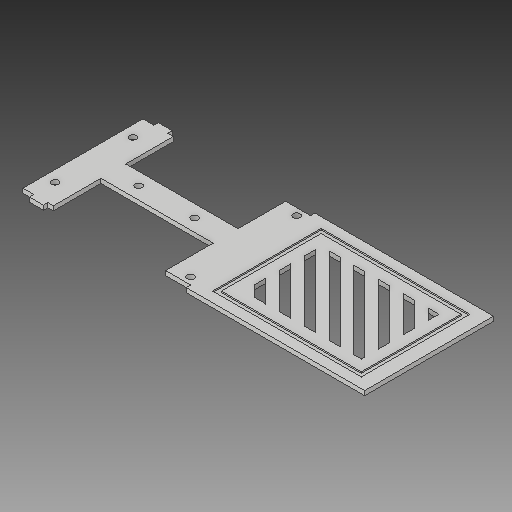
# Autodesk Inventor part: cuerpo-base-bateria
Saved by Autodesk Inventor 2019 (Build 230136000, 136)
## iProperties
Created: 2020-03-02
Part Number: cuerpo-base-bateria
Material: Generic
Document SubType Name: Modeling
Designer: jacqu
Density: 1 g/cm^3
Appearance: Default
ancho_acople_hombros: 86.662 mm
largo_abdomen_robot: 146.950 mm
Author: jacqu
Autodesk Inventor part; units mm, degrees
ref_plane "YZ Plane" through (0, 0, 0) normal (1, 0, 0) x (0, 1, 0)
ref_plane "XZ Plane" through (0, 0, 0) normal (0, 1, 0) x (-1, 0, 0)
ref_plane "XY Plane" through (0, 0, 0) normal (0, 0, 1) x (1, 0, 0)
sketch "Sketch9" plane through (0, 0, 0) normal (0, 1, 0) x (-1, 0, 0)
  line L0 (0, 0) -> (-250, 0)
  line L1 (-250, 0) -> (-250, -86.6623)
  line L2 (-250, -86.6623) -> (0, -86.6623)
  line L3 (0, -86.6623) -> (0, 0)
  dimension "d59" = 86.6623
  dimension "d60" = 250
  constraints: 8 end point, 2 parallel, 1 horizontal, 1 perpendicular
  measures "d59" distance of L2.end L0.start
  measures "d60" distance between parallel lines of L3 L1
extrude "Extrusion5" add sketch "Sketch9" along normal blind 3.2
sketch "Sketch10" plane through (0, 3.2, 0) normal (0, 1, 0) x (1, 0, 0)
  line L0 (22, 0) -> (103.05, 0)
  line L1 (103.05, 0) -> (103.05, 34.3311)
  line L2 (103.05, 34.3311) -> (22, 34.3311)
  line L3 (22, 34.3311) -> (22, 0)
  line L4 (250, 86.6623) -> (0, 86.6623) projected
  line L5 (103.05, 86.6623) -> (22, 86.6623)
  line L6 (22, 86.6623) -> (22, 52.3311)
  line L7 (22, 52.3311) -> (103.05, 52.3311)
  line L8 (103.05, 52.3311) -> (103.05, 86.6623)
  line L9 (0, 0) -> (250, 0) projected
  line L10 (0, 86.6623) -> (0, 0) projected
  dimension "d63" = 22
  dimension "d64" = 34.3311
  dimension "d65" = 81.05
  dimension "d66" = 34.3311
  constraints: 16 end point, 4 parallel, 4 point on line, 2 horizontal, 2 perpendicular
  measures "d63" distance between parallel lines of L10 L3
  measures "d64" distance of L2.end L0.start
  measures "d65" distance between parallel lines of L3 L1
  measures "d66" distance between parallel lines of L4 L7
extrude "Extrusion6" cut sketch "Sketch10" against normal blind 3.2
sketch "Sketch11" plane through (0, 3.2, 0) normal (0, 1, 0) x (1, 0, 0)
  line L0 (237.05, 7.3311) -> (136.05, 7.3311)
  line L1 (136.05, 7.3311) -> (136.05, 79.3311)
  line L2 (136.05, 79.3311) -> (237.05, 79.3311)
  line L3 (237.05, 79.3311) -> (237.05, 7.3311)
  line L4 (103.05, 86.6623) -> (103.05, 52.3311) projected
  line L5 (0, 86.6623) -> (0, 0) projected
  line L6 (103.05, 0) -> (250, 0) projected
  line L7 (121.05, 0) -> (121.05, 86.188) construction
  line L8 (103.05, 34.3311) -> (103.05, 0) projected
  line L9 (240.25, 4.1311) -> (132.85, 4.1311)
  line L10 (132.85, 4.1311) -> (132.85, 82.5311)
  line L11 (132.85, 82.5311) -> (240.25, 82.5311)
  line L12 (240.25, 82.5311) -> (240.25, 4.1311)
  dimension "d69" = 72
  dimension "d70" = 101
  dimension "d71" = 33
  dimension "d72" = 86.6623
  dimension "d73" = 7.3311
  dimension "d74" = 18
  dimension "d75" = 3.2
  dimension "d76" = 3.2
  dimension "d77" = 3.2
  dimension "d78" = 3.2
  constraints: 18 end point, 4 parallel, 2 horizontal, 2 perpendicular, 1 point on line, 1 vertical
  measures "d69" distance of L2.end L0.start
  measures "d70" distance of L1.end L2.end
  measures "d71" distance between parallel lines of L4 L1
  measures "d72" distance of L5.start L5.end
  measures "d73" distance between parallel lines of L6 L0
  measures "d74" distance between parallel lines of L7 L8
  measures "d75" distance between parallel lines of L3 L12
  measures "d76" distance between parallel lines of L9 L0
  measures "d77" distance between parallel lines of L11 L2
  measures "d78" distance between parallel lines of L10 L1
extrude "Extrusion7" cut sketch "Sketch11" against normal blind 1
sketch "Sketch12" plane through (0, 3.2, 0) normal (0, 1, 0) x (1, 0, 0)
  line L0 (237.05, 7.3311) -> (237.05, 79.3311) projected
  line L1 (237.05, 79.3311) -> (136.05, 79.3311) projected
  line L2 (136.05, 79.3311) -> (136.05, 7.3311) construction
  line L3 (136.05, 7.3311) -> (237.05, 7.3311) projected
  line L4 (144.05, 15.3311) -> (229.05, 15.3311) construction
  line L5 (229.05, 15.3311) -> (229.05, 71.3311) construction
  line L6 (229.05, 71.3311) -> (144.05, 71.3311) construction
  line L7 (144.05, 71.3311) -> (144.05, 15.3311) construction
  line L8 (152.05, 15.3311) -> (144.05, 23.3311)
  line L9 (144.05, 23.3311) -> (144.05, 31.3311)
  line L10 (144.05, 31.3311) -> (160.05, 15.3311)
  line L11 (160.05, 15.3311) -> (152.05, 15.3311)
  line L12 (169.9495, 15.3311) -> (144.05, 41.2306)
  line L13 (144.05, 41.2306) -> (144.05, 49.2306)
  line L14 (144.05, 49.2306) -> (177.9495, 15.3311)
  line L15 (169.9495, 15.3311) -> (177.9495, 15.3311)
  line L16 (187.849, 15.3311) -> (144.05, 59.1301)
  line L17 (144.05, 59.1301) -> (144.05, 67.1301)
  line L18 (144.05, 67.1301) -> (195.849, 15.3311)
  line L19 (195.849, 15.3311) -> (187.849, 15.3311)
  line L20 (213.7485, 15.3311) -> (205.7485, 15.3311)
  line L21 (157.7485, 71.3311) -> (213.7485, 15.3311)
  line L22 (223.648, 15.3311) -> (167.648, 71.3311)
  line L23 (185.5475, 71.3311) -> (193.5475, 71.3311)
  line L24 (193.5475, 71.3311) -> (229.05, 35.8286)
  line L25 (229.05, 45.7281) -> (203.447, 71.3311)
  line L26 (203.447, 71.3311) -> (211.447, 71.3311)
  line L27 (229.05, 63.6276) -> (221.3465, 71.3311)
  line L28 (229.05, 45.7281) -> (229.05, 53.7281)
  line L29 (229.05, 53.7281) -> (211.447, 71.3311)
  line L30 (205.7485, 15.3311) -> (149.7485, 71.3311)
  line L31 (149.7485, 71.3311) -> (157.7485, 71.3311)
  line L32 (185.5475, 71.3311) -> (229.05, 27.8286)
  line L33 (229.05, 27.8286) -> (229.05, 35.8286)
  line L34 (223.648, 15.3311) -> (229.05, 15.3311)
  line L35 (229.05, 15.3311) -> (229.05, 17.9291)
  line L36 (229.05, 17.9291) -> (175.648, 71.3311)
  line L37 (167.648, 71.3311) -> (175.648, 71.3311)
  line L38 (229.05, 63.6276) -> (229.05, 71.3311)
  line L39 (229.05, 71.3311) -> (221.3465, 71.3311)
  point P0 (0, 0)
  dimension "d81" = 8
  dimension "d82" = 8
  dimension "d83" = 8
  dimension "d84" = 8
  dimension "d85" = 8
  dimension "d86" = 8
  dimension "d88" = 7
  dimension "d90" = 7
  dimension "d92" = 7
  dimension "d95" = 7
  dimension "d97" = 7
  dimension "d98" = 7
  dimension "d100" = 7
  constraints: 66 end point, 12 parallel, 8 equal length, 6 point on line, 5 horizontal, 2 perpendicular, 2 vertical, 33 other
  measures "d81" distance between parallel lines of L2 L7
  measures "d85" distance of L7.end L8.end
  measures "d86" distance of L12.end L13.end
  measures "d88" distance between parallel lines of L16 L14
  measures "d90" distance between parallel lines of L22 L21
  measures "d92" distance between parallel lines of L25 L24
  measures "d95" distance between parallel lines of L12 L10
  measures "d97" distance between parallel lines of L27 L29
  measures "d98" distance between parallel lines of L30 L18
  measures "d100" distance between parallel lines of L32 L36
extrude "Extrusion8" cut sketch "Sketch12" against normal up to surface (3.2 mm away)
sketch "Sketch13" plane through (0, 3.2, 0) normal (0, 1, 0) x (1, 0, 0)
  circle A0 centre (116.05, 5) radius 2.5
  circle A1 centre (116.05, 81.6623) radius 2.5
  circle A2 centre (40.35, 43.3311) radius 2.5
  circle A3 centre (80.7, 43.3311) radius 2.5
  line L0 (0, 86.6623) -> (0, 0) projected
  line L1 (103.05, 0) -> (250, 0) projected
  line L2 (103.05, 34.3311) -> (103.05, 0) projected
  line L3 (250, 86.6623) -> (103.05, 86.6623) projected
  circle A4 centre (8, 15.25) radius 2.5
  circle A5 centre (8, 71.4123) radius 2.5
  line L4 (0, 0) -> (22, 0) projected
  line L5 (22, 86.6623) -> (0, 86.6623) projected
  point P0 (0, 43.3311)
  dimension "d103" = 40.35
  dimension "d104" = 40.35
  dimension "d105" = 5
  dimension "d106" = 5
  dimension "d107" = 13
  dimension "d108" = 5
  dimension "d109" = 15.25
  dimension "d110" = 15.25
  dimension "d111" = 8
  constraints: 6 centre point, 5 equal radius, 2 horizontal alignment, 2 vertical alignment, 1 midpoint
  measures "d103" distance from line of A2.centre L0
  measures "d104" distance of A3.centre A2.centre
  measures "d105" diameter of A2
  measures "d106" distance from line of L1 A0.centre
  measures "d107" distance from line of L2 A0.centre
  measures "d108" distance from line of L3 A1.centre
  measures "d109" distance from line of L4 A4.centre
  measures "d110" distance from line of L5 A5.centre
  measures "d111" distance from line of L0 A5.centre
extrude "Extrusion9" cut sketch "Sketch13" against normal up to surface (3.2 mm away)
sketch "Sketch14" plane through (0, 3.2, 0) normal (0, 1, 0) x (1, 0, 0)
  line L0 (250, 0) -> (250, 86.6623) projected
  line L1 (103.05, 34.3311) -> (103.05, 0) projected
  point P0 (0, 0)
  dimension "largo_abdomen_robot" = 146.95
  measures "largo_abdomen_robot" distance between parallel lines of L0 L1
sketch "Sketch15" plane through (0, 3.2, 0) normal (0, 1, 0) x (1, 0, 0)
  line L0 (250, 0) -> (250, 86.6623) projected
  line L1 (250, 86.6623) -> (121.05, 86.6623)
  line L2 (121.05, 86.6623) -> (121.05, 89.8623)
  line L3 (121.05, 89.8623) -> (250, 89.8623)
  line L4 (250, 89.8623) -> (250, 86.6623)
  line L5 (250, 0) -> (121.05, 0)
  line L6 (121.05, 0) -> (121.05, -3.2)
  line L7 (121.05, -3.2) -> (250, -3.2)
  line L8 (250, -3.2) -> (250, 0)
  point P0 (0, 0)
  dimension "d115" = 128.95
  dimension "d116" = 3.2
  constraints: 16 end point, 4 parallel, 2 horizontal, 2 perpendicular, 1 collinear, 1 point on line
  measures "d115" distance of L2.end L3.end
  measures "d116" distance between parallel lines of L3 L1
extrude "Extrusion10" add sketch "Sketch15" against normal up to surface (3.2 mm away)
sketch "Sketch16" plane through (0, 3.2, 0) normal (0, 1, 0) x (1, 0, 0)
  line L0 (0, 0) -> (22, 0) projected
  line L1 (18, 0) -> (8, 0)
  line L2 (8, 0) -> (8, -3.2)
  line L3 (8, -3.2) -> (18, -3.2)
  line L4 (18, -3.2) -> (18, 0)
  line L5 (18, 86.6623) -> (8, 86.6623)
  line L6 (8, 86.6623) -> (8, 89.8623)
  line L7 (8, 89.8623) -> (18, 89.8623)
  line L8 (18, 89.8623) -> (18, 86.6623)
  line L9 (22, 86.6623) -> (0, 86.6623) projected
  line L10 (22, 0) -> (22, 34.3311) projected
  dimension "d119" = 4
  dimension "d120" = 10
  dimension "d121" = 3.2
  constraints: 16 end point, 4 parallel, 4 point on line, 2 horizontal, 2 perpendicular, 1 collinear
  measures "d119" distance between parallel lines of L4 L10
  measures "d120" distance of L2.end L3.end
  measures "d121" distance of L1.end L2.end
extrude "Extrusion11" add sketch "Sketch16" against normal up to surface (3.2 mm away)
equation "\"d59\" = ancho_acople_hombros"
equation "\"d63\" = acople_hombro_grosor_frontal"
equation "\"d64\" = acople_hombro_ancho_agujero"
equation "\"d65\" = acople_hombro_largo_agujero"
equation "\"d66\" = acople_hombro_ancho_agujero"
equation "\"d73\" = -0.5 * d69 + 0.5 * d72"
equation "\"d74\" = acople_hombro_grosor_trasero"
equation "\"d76\" = d75"
equation "\"d77\" = d76"
equation "\"d78\" = d75"
equation "\"d82\" = d81"
equation "\"d83\" = d81"
equation "\"d84\" = d81"
equation "\"d86\" = d85"
equation "\"d88\" = d95"
equation "\"d90\" = d95"
equation "\"d92\" = d91"
equation "\"d97\" = d92"
equation "\"d98\" = d95"
equation "\"d100\" = d95"
equation "\"d103\" = dist_agujero_central_a_frente"
equation "\"d104\" = d103"
equation "\"d105\" = diametro_tornillo"
equation "\"d106\" = dist_agujero_trasero_a_lado"
equation "\"d107\" = dist_agujero_trasero_a_frente"
equation "\"d108\" = d106"
equation "\"d109\" = dist_agujero_frontal_a_lateral"
equation "\"d110\" = d109"
equation "\"d111\" = dist_agujero_frontal_a_frente"
equation "\"d115\" = largo_abdomen_robot - acople_hombro_grosor_trasero"
equation "\"d91\" = d90"
equation "\"ancho_acople_hombros\" = 86.662258"
equation "\"acople_hombro_grosor_frontal\" = 22"
equation "\"acople_hombro_ancho_agujero\" = 34.331129"
equation "\"acople_hombro_largo_agujero\" = 81.05"
equation "\"acople_hombro_grosor_trasero\" = 18"
equation "\"dist_agujero_central_a_frente\" = 40.35"
equation "\"diametro_tornillo\" = 5"
equation "\"dist_agujero_trasero_a_lado\" = 5"
equation "\"dist_agujero_trasero_a_frente\" = 13"
equation "\"dist_agujero_frontal_a_lateral\" = 15.25"
equation "\"dist_agujero_frontal_a_frente\" = 8"
body "Solid3"
